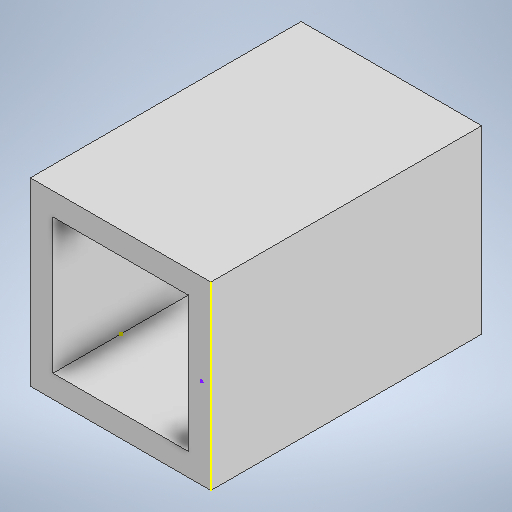
# Autodesk Inventor part: Peça6_cube
Saved by Autodesk Inventor 2025.2 (Build 292293000, 293)
## iProperties
Created: 2025-03-26
Part Number: Peça6_cube
Material: Genérico
Document SubType Name: Modeling
Designer: Formação
Density: 1 g/cm^3
Appearance: Padrão
Author: Formação
Autodesk Inventor part; units mm, degrees
ref_plane "YZ Plane" through (0, 0, 0) normal (1, 0, 0) x (0, 1, 0)
ref_plane "XZ Plane" through (0, 0, 0) normal (0, 1, 0) x (-1, 0, 0)
ref_plane "XY Plane" through (0, 0, 0) normal (0, 0, 1) x (1, 0, 0)
sketch "Esboço1" plane through (0, 0, 0) normal (0, 0, 1) x (1, 0, 0)
  line L0 (-10, 10) -> (10, 10)
  line L1 (10, 10) -> (10, -10)
  line L2 (10, -10) -> (-10, -10)
  line L3 (-10, -10) -> (-10, 10)
  line L4 (-10, 10) -> (10, -10) construction
  line L5 (10, 10) -> (-10, -10) construction
  line L6 (-7.5, -7.5) -> (7.5, -7.5)
  line L7 (7.5, -7.5) -> (7.5, 7.5)
  line L8 (7.5, 7.5) -> (-7.5, 7.5)
  line L9 (-7.5, 7.5) -> (-7.5, -7.5)
  line L10 (-7.5, -7.5) -> (7.5, 7.5) construction
  line L11 (7.5, -7.5) -> (-7.5, 7.5) construction
  point P0 (0, 0)
  point P1 (0, 0)
  point P2 (0, 0)
  dimension "d0" = 20
  dimension "d1" = 10
  dimension "d2" = 15
  dimension "d3" = 15
  constraints: 24 end point, 4 coincident, 4 midpoint, 4 parallel, 2 horizontal, 2 perpendicular
  measures "d0" distance of L1.end L0.end
  measures "d1" horizontal distance of L2.end point (0, 0)
  measures "d2" distance of L8.end L7.end
  measures "d3" distance of L7.end L6.end
extrude "Extrusão1" add sketch "Esboço1" along normal mid plane 30
sketch "Esboço2" plane through (0, 0, 15) normal (0, 0, 1) x (1, 0, 0)
  line L0 (10, -10) -> (10, 10) projected
  point P0 (0, 0)
  point P1 (9, 0)
sketch "Esboço10" plane through (0, 0, 0) normal (1, 0, 0) x (0, 1, 0)
  point P0 (0, 0)
sketch "Esboço12" plane through (0, 0, 0) normal (1, 0, 0) x (0, 1, 0)
  line L0 (9, 14) -> (7, 14)
  line L1 (7, 14) -> (7, 12)
  line L2 (7, 12) -> (9, 12)
  line L3 (9, 12) -> (9, 14)
  line L4 (9, 14) -> (7, 12) construction
  line L5 (7, 14) -> (9, 12) construction
  point P0 (0, 0)
  point P1 (8, 13)
  constraints: 12 end point, 2 midpoint, 2 parallel, 1 horizontal, 1 perpendicular
